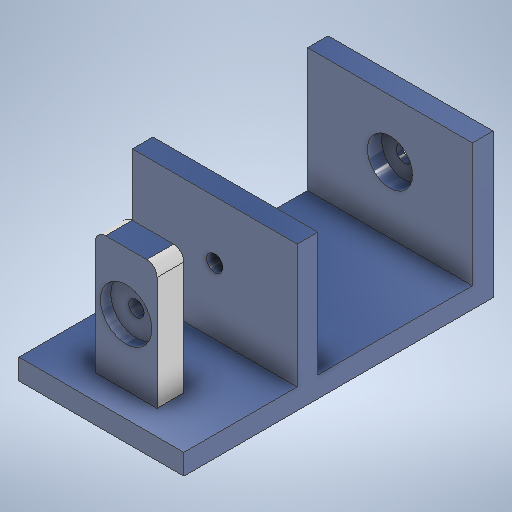
# Autodesk Inventor part: soporte_inferior
Saved by Autodesk Inventor 2026 (Build 300175050, 175E)
## iProperties
Created: 2025-06-30
Part Number: soporte_inferior
Material: Genérico
Document SubType Name: Modeling
Designer: piero
Density: 1 g/cm^3
Appearance: Valor por defecto
Author: piero
Autodesk Inventor part; units mm, degrees
ref_plane "YZ Plane" through (0, 0, 0) normal (1, 0, 0) x (0, 1, 0)
ref_plane "XZ Plane" through (0, 0, 0) normal (0, 1, 0) x (-1, 0, 0)
ref_plane "XY Plane" through (0, 0, 0) normal (0, 0, 1) x (1, 0, 0)
sketch "Boceto1" plane through (0, 0, 0) normal (0, 1, 0) x (-1, 0, 0)
  line L0 (0, 0) -> (80, 0)
  line L1 (80, 0) -> (80, -150)
  line L2 (80, -150) -> (0, -150)
  line L3 (0, -150) -> (0, 0)
  line L4 (80, -150) -> (0, -150)
  line L5 (0, -150) -> (0, -140)
  line L6 (0, -140) -> (80, -140)
  line L7 (80, -140) -> (80, -150)
  line L8 (80, -65) -> (0, -65)
  line L9 (0, -65) -> (0, -55)
  line L10 (0, -55) -> (80, -55)
  line L11 (80, -55) -> (80, -65)
  line L12 (80, -25) -> (0, -25)
  line L13 (0, -25) -> (0, -12)
  line L14 (0, -12) -> (80, -12)
  line L15 (80, -12) -> (80, -25)
  point P0 (0, -65)
  point P1 (0, -12)
  point P2 (80, -12)
  point P3 (0, -25)
  point P4 (0, -55)
  point P5 (80, -55)
  dimension "d0" = 80
  dimension "d1" = 150
  dimension "d4" = 80
  dimension "d5" = 10
  dimension "d6" = 80
  dimension "d7" = 10
  dimension "d8" = 80
  dimension "d9" = 13
  dimension "d17" = 75
  dimension "d19" = 30
  constraints: 32 end point, 8 parallel, 4 horizontal, 4 perpendicular, 2 point on line
  measures "d0" distance of L1.end L2.end
  measures "d1" distance of L0.end L1.end
  measures "d4" distance of L5.end L6.end
  measures "d5" distance of L4.end L5.end
  measures "d6" distance of L9.end L10.end
  measures "d7" distance of L8.end L9.end
  measures "d8" distance of L13.end L14.end
  measures "d9" distance of L12.end L13.end
  measures "d17" distance between parallel lines of L8 L6
  measures "d19" distance between parallel lines of L10 L12
extrude "Extrusión1" add sketch "Boceto1" along normal blind 10 contours L0 L1 L14 L3 | L12 L1 L10 L3 | L8 L1 L6 L3
extrude "Extrusión2" add sketch "Boceto1" along normal blind 70 contours L14 L1 L12 L3 | L10 L1 L8 L3 | L6 L1 L2 L3
sketch "Boceto3" plane through (0, 0, -150) normal (0, 0, -1) x (-1, 0, 0)
  circle A0 centre (40, 42) radius 4
  line L0 (0, 0) -> (0, 70) projected
  line L1 (0, 70) -> (80, 70) projected
  line L2 (80, 10) -> (0, 10) projected
  circle A1 centre (40, 42) radius 11
  dimension "d12" = 8
  dimension "d13" = 40
  dimension "d18" = 32
  dimension "d54" = 22
  constraints: 2 centre point, 1 coincident
  measures "d12" diameter of A0
  measures "d13" distance from line of A0.centre L0
  measures "d18" distance from line of L2 A0.centre
  measures "d54" diameter of A1
extrude "Extrusión3" cut sketch "Boceto3" against normal blind 10 contours A0
sketch "Boceto4" plane through (-80, 10, -12) normal (0, 0, 1) x (1, 0, 0)
  circle A0 centre (40, 32) radius 4 projected
  circle A1 centre (40, 32) radius 3.75
  circle A2 centre (40, 32) radius 12.5
  point P0 (80, -10)
  dimension "d20" = 7.5
  dimension "d21" = 25
  constraints: 2 centre point, 2 coincident
  measures "d20" diameter of A1
  measures "d21" diameter of A2
extrude "Extrusión4" cut sketch "Boceto4" against normal blind 10 contours A1
extrude "Extrusión6" cut sketch "Boceto4" against normal blind 5 contours A0 | A2
sketch "Boceto5" plane through (0, 10, -65) normal (0, 0, -1) x (-1, 0, 0)
  circle A0 centre (40, 32) radius 3.75 projected
  circle A1 centre (40, 32) radius 4
  point P0 (0, -10)
  dimension "d44" = 8
  constraints: 1 centre point, 1 coincident
  measures "d44" diameter of A1
extrude "Extrusión7" cut sketch "Boceto5" against normal blind 10 contours A0 | A1
sketch "Boceto6" plane through (-80, 10, -140) normal (0, 0, 1) x (1, 0, 0)
  circle A0 centre (40, 32) radius 3.75 projected
  circle A1 centre (40, 32) radius 11
  point P0 (80, -10)
  dimension "d55" = 22
  constraints: 1 centre point, 1 coincident
  measures "d55" diameter of A1
extrude "Extrusión8" cut sketch "Boceto6" against normal blind 7
fillet "Empalme1" radius 20 1 edges at (0, 70, -18.5)
fillet "Empalme2" radius 20 1 edges at (-80, 70, -18.5)
sketch "Boceto7" plane through (-80, 10, -12) normal (0, 0, 1) x (1, 0, 0)
  line L0 (0, 0) -> (80, 0) projected
  line L1 (20, 60) -> (60, 60) projected
  line L2 (0, 0) -> (25, 0)
  line L3 (25, 0) -> (25, 60)
  line L4 (25, 60) -> (0, 60)
  line L5 (0, 60) -> (0, 0)
  line L6 (80, 0) -> (80, 40) projected
  line L7 (80, 0) -> (55, 0)
  line L8 (55, 0) -> (55, 60)
  line L9 (55, 60) -> (80, 60)
  line L10 (80, 60) -> (80, 0)
  point P0 (80, -10)
  point P1 (60, 60)
  point P2 (55, 60)
  point P3 (55, 0)
  point P4 (25, 0)
  point P5 (20, 60)
  dimension "d60" = 25
  dimension "d61" = 25
  constraints: 16 end point, 4 parallel, 2 horizontal, 2 perpendicular, 2 point on line
  measures "d60" distance of L4.end L3.end
  measures "d61" distance of L8.end L9.end
extrude "Extrusión9" cut sketch "Boceto7" against normal blind 13 contours L5 L4 L1 L3 L0 | L8 L1 L9 L10 L6 L0
fillet "Empalme3" radius 5 1 edges at (-25, 70, -18.5)
fillet "Empalme4" radius 5 1 edges at (-55, 70, -18.5)
